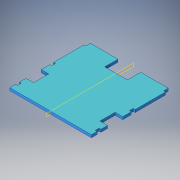
# Autodesk Inventor part: RhinoBottomFloorPlate01-ExtendedBy3Inches
Saved by Autodesk Inventor 2016 SP1 (Build 200210100, 210)
## iProperties
Created: 2015-12-30
Part Number: RhinoBottomFloorPlate01-ExtendedBy3Inches
Material: Wood (Birch)
Document SubType Name: Modeling
Designer: steele
Density: 0.55 g/cm^3
Appearance: Cyan
Mass: 2038.6 g
Surface Area: 4559.99 cm^2
Volume: 3706.55 cm^3
Author: steele
Autodesk Inventor part; units mm, degrees
ref_plane "XZ Plane" through (0, 0, 0) normal (0, 1, 0) x (-1, 0, 0)
ref_plane "XY Plane" through (0, 0, 0) normal (0, 0, 1) x (1, 0, 0)
sketch "Sketch1" plane through (0, 0, 0) normal (0, 1, 0) x (-1, 0, 0)
  line L0 (-273.05, 263.525) -> (-273.05, -263.525)
  line L1 (-273.05, -263.525) -> (273.05, -263.525)
  line L2 (273.05, -263.525) -> (273.05, 263.525)
  line L3 (273.05, 263.525) -> (-273.05, 263.525)
  line L4 (-273.05, 263.525) -> (273.05, -263.525) construction
  line L5 (-273.05, -263.525) -> (273.05, 263.525) construction
  point P0 (0, 0)
  dimension "baseLength" = 527.05
  dimension "baseWidth" = 546.1
  constraints: 12 end point, 2 midpoint, 2 parallel, 1 perpendicular, 1 vertical
  measures "baseLength" distance of L0.start L0.end
  measures "baseWidth" distance of L2.end L0.start
extrude "Extrusion1" add sketch "Sketch1" along normal blind 17.78
sketch "Sketch2" plane through (0, 0, 0) normal (0, -1, 0) x (1, 0, 0)
  line L0 (273.05, 263.525) -> (273.05, -263.525) projected
  line L1 (273.05, 155.575) -> (222.25, 155.575)
  line L2 (222.25, 155.575) -> (222.25, 53.975)
  line L3 (222.25, 53.975) -> (273.05, 53.975)
  line L4 (273.05, 53.975) -> (273.05, 155.575)
  line L5 (-273.05, 263.525) -> (273.05, 263.525) projected
  point P0 (0, 0)
  dimension "backToEndOfGearBox" = 107.95
  dimension "backToFrontOfGearBox" = 209.55
  dimension "wdithForGearBox" = 50.8
  constraints: 8 end point, 2 perpendicular, 2 point on line, 1 collinear, 1 horizontal
  measures "backToEndOfGearBox" distance between parallel lines of L1 L5
  measures "backToFrontOfGearBox" distance between parallel lines of L3 L5
  measures "wdithForGearBox" distance between parallel lines of L2 L0
extrude "Extrusion2" cut sketch "Sketch2" against normal through all
mirror "Mirror1" about plane through (0, 0, 0) normal (1, 0, 0) of "Extrusion2"
sketch "Sketch3" plane through (0, 17.78, 0) normal (0, 1, 0) x (1, 0, 0)
  line L0 (273.05, -225.425) -> (260.35, -225.425)
  line L1 (260.35, -225.425) -> (260.35, -200.025)
  line L2 (260.35, -200.025) -> (273.05, -200.025)
  line L3 (273.05, -200.025) -> (273.05, -225.425)
  line L4 (273.05, -263.525) -> (273.05, -155.575) projected
  line L5 (-273.05, -263.525) -> (273.05, -263.525) projected
  point P0 (0, 0)
  dimension "d9" = 25.4
  dimension "d10" = 12.7
  dimension "d11" = 38.1
  constraints: 8 end point, 2 parallel, 1 collinear, 1 horizontal, 1 perpendicular
  measures "d9" distance of L0.end L1.end
  measures "d10" distance of L0.start L0.end
  measures "d11" distance between parallel lines of L0 L5
extrude "Extrusion3" cut sketch "Sketch3" against normal through all
mirror "Mirror2" about plane through (0, 0, 0) normal (1, 0, 0) of "Extrusion3"
sketch "Sketch4" plane through (0, 17.78, 0) normal (0, 1, 0) x (1, 0, 0)
  line L0 (273.05, -53.975) -> (273.05, 263.525) projected
  line L1 (273.05, 3.175) -> (260.35, 3.175)
  line L2 (260.35, 3.175) -> (260.35, 28.575)
  line L3 (260.35, 28.575) -> (273.05, 28.575)
  line L4 (273.05, 28.575) -> (273.05, 3.175)
  line L5 (-273.05, -263.525) -> (273.05, -263.525) projected
  point P0 (0, 0)
  dimension "d14" = 25.4
  dimension "d15" = 266.7
  dimension "d16" = 12.7
  constraints: 8 end point, 2 parallel, 1 horizontal, 1 perpendicular, 1 point on line
  measures "d14" distance of L1.end L2.end
  measures "d15" distance between parallel lines of L1 L5
  measures "d16" distance of L1.start L1.end
extrude "Extrusion4" cut sketch "Sketch4" against normal through all
mirror "Mirror3" about plane through (0, 0, 0) normal (1, 0, 0) of "Extrusion4"
sketch "Sketch5" plane through (0, 17.78, 0) normal (0, 1, 0) x (1, 0, 0)
  line L0 (273.05, 231.775) -> (260.35, 231.775)
  line L1 (260.35, 231.775) -> (260.35, 263.525)
  line L2 (260.35, 263.525) -> (273.05, 263.525)
  line L3 (273.05, 263.525) -> (273.05, 231.775)
  line L4 (273.05, 28.575) -> (273.05, 263.525) projected
  line L5 (273.05, 263.525) -> (-273.05, 263.525) projected
  point P0 (0, 0)
  dimension "d19" = 12.7
  dimension "d20" = 31.75
  constraints: 8 end point, 2 collinear, 2 parallel, 1 horizontal, 1 perpendicular
  measures "d19" distance of L0.start L0.end
  measures "d20" distance between parallel lines of L0 L5
extrude "Extrusion5" cut sketch "Sketch5" against normal through all
mirror "Mirror4" about plane through (0, 0, 0) normal (1, 0, 0) of "Extrusion5"
sketch "Sketch8" plane through (0, 17.78, 0) normal (0, 1, 0) x (1, 0, 0)
  line L0 (-76.2, 263.525) -> (76.2, 263.525)
  line L1 (76.2, 263.525) -> (76.2, 174.625)
  line L2 (76.2, 174.625) -> (-76.2, 174.625)
  line L3 (-76.2, 174.625) -> (-76.2, 263.525)
  line L4 (260.35, 263.525) -> (-260.35, 263.525) projected
  point P0 (0, 0)
  dimension "d23" = 76.2
  dimension "d24" = 76.2
  dimension "d25" = 88.9
  constraints: 8 end point, 2 parallel, 1 collinear, 1 horizontal, 1 perpendicular
  measures "d23" distance from line of point (0, 0) L3
  measures "d24" distance from line of point (0, 0) L1
  measures "d25" distance between parallel lines of L2 L0
extrude "Extrusion6" cut sketch "Sketch8" against normal through all
equation "\"baseLength\" = userBaseLength"
equation "\"baseWidth\" = userBaseWidth"
equation "\"d9\" = lengthOfSpacingForBolt"
equation "\"d10\" = widthOfSpacingForBolt"
equation "\"d11\" = distanceFromBackForEndBolt"
equation "\"d14\" = lengthOfSpacingForBolt"
equation "\"d16\" = widthOfSpacingForBolt"
equation "\"d19\" = widthOfSpacingForBolt"
equation "\"spaceingAlongSides\" = 3.175"
equation "\"distanceFromBackForEndBolt\" = 38.1"
equation "\"widthOfSpacingForBolt\" = 12.7"
equation "\"lengthOfSpacingForBolt\" = 25.4"
equation "\"userBaseLength\" = 527.05"
equation "\"userBaseWidth\" = 546.1"
body "Solid1"
